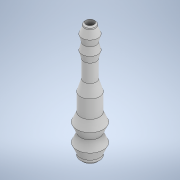
# Autodesk Inventor part: Barbed to Barbed 4mm ID to 2.4mm ID
Saved by Autodesk Inventor 2021 (Build 250183000, 183)
## iProperties
Created: 2020-12-17
Part Number: Barbed to Barbed 4mm ID to 2.4mm ID
Material: Generic
Document SubType Name: Modeling
Designer: natha
Density: 1 g/cm^3
Appearance: Default
Author: natha
Autodesk Inventor part; units mm, degrees
ref_plane "YZ Plane" through (0, 0, 0) normal (1, 0, 0) x (0, 1, 0)
ref_plane "XZ Plane" through (0, 0, 0) normal (0, 1, 0) x (-1, 0, 0)
ref_plane "XY Plane" through (0, 0, 0) normal (0, 0, 1) x (1, 0, 0)
sketch "Sketch1" plane through (0, 0, 0) normal (0, 0, 1) x (1, 0, 0)
  line L0 (-0.9, 16.5) -> (-0.9, -5.2047)
  line L1 (0, 21.8) -> (0, -15.3) construction
  line L2 (-0.9, 16.5) -> (-1.2, 16.2)
  line L3 (-1.2, 16.2) -> (-1.2, 15.9)
  line L4 (-1.2, 15.9) -> (-1.8, 14.3)
  line L5 (-1.8, 14.3) -> (-1.4, 12.7)
  line L6 (-1.4, 12.7) -> (-1.8, 11.1)
  line L7 (-1.8, 11.1) -> (-1.4, 9.5)
  line L8 (-1.4, 9.5) -> (-1.4, 5.5)
  line L9 (-1.4, 5.5) -> (-2.15, 3)
  line L10 (-2.15, 3) -> (-2.15, -1)
  line L11 (-2.15, -1) -> (-3, -3)
  line L12 (-3, -3) -> (-2.15, -5)
  line L13 (-2.15, -5) -> (-3, -7)
  line L14 (-3, -7) -> (-2.15, -9)
  line L15 (-2.15, -9) -> (-2.15, -9.5)
  line L16 (-2.15, -9.5) -> (-1.65, -10)
  line L17 (-1.65, -10) -> (-0.9, -10)
  line L18 (-0.9, -10) -> (-0.9, -5.2047)
  line L19 (-3.42, 0) -> (-0.48, 0) construction
  dimension "d5" = 0.9
  dimension "d6" = 1.8
  dimension "d15" = 1.2
  dimension "d16" = 1.8
  dimension "d18" = 45
  dimension "d19" = 0.3
  dimension "d20" = 1.4
  dimension "d21" = 1.4
  dimension "d22" = 1.6
  dimension "d23" = 1.6
  dimension "d24" = 1.6
  dimension "d27" = 4
  dimension "d29" = 2.5
  dimension "d30" = 2.15
  dimension "d31" = 4
  dimension "d32" = 1.6
  dimension "d33" = 2
  dimension "d34" = 2
  dimension "d35" = 2
  dimension "d36" = 2
  dimension "d37" = 3
  dimension "d38" = 2.15
  dimension "d39" = 3
  dimension "d41" = 45
  dimension "d42" = 0.5
  dimension "d43" = 0.5
  dimension "d44" = 10
  constraints: 36 end point, 4 vertical, 1 collinear, 1 parallel, 1 perpendicular
  measures "d5" distance between parallel lines of L1 L0
  measures "d6" distance from line of L1 L4.end
  measures "d15" distance between parallel lines of L1 L3
  measures "d16" distance from line of L1 L6.end
  measures "d18" angle of L1 L2
  measures "d19" distance of L2.end L3.end
  measures "d20" distance from line of L1 L5.end
  measures "d21" distance from line of L1 L7.end
  measures "d22" vertical distance of L4.end L3.end
  measures "d23" vertical distance of L7.end L6.end
  measures "d24" vertical distance of L6.end L5.end
  measures "d27" distance of L7.end L8.end
  measures "d29" vertical distance of L8.end L9.end
  measures "d30" distance from line of L1 L9.end
  measures "d31" distance of L9.end L10.end
  measures "d32" vertical distance of L5.end L4.end
  measures "d33" vertical distance of L10.end L11.end
  measures "d34" vertical distance of L11.end L12.end
  measures "d35" vertical distance of L12.end L13.end
  measures "d36" vertical distance of L13.end L14.end
  measures "d37" distance from line of L1 L11.end
  measures "d38" distance from line of L1 L12.end
  measures "d39" distance from line of L1 L13.end
  measures "d41" angle of L1 L16
  measures "d42" horizontal distance of L16.end L15.end
  measures "d43" distance of L14.end L15.end
  measures "d44" distance between parallel lines of L19 L17
revolve "Revolution1" add sketch "Sketch1" angle 360 about axis through (0, 0, 0) along (0, -1, 0)
equation "\"d23\" = d22"
equation "\"d24\" = d22"
equation "\"d32\" = d22"
equation "\"d34\" = d33"
equation "\"d35\" = d33"
equation "\"d36\" = d33"
equation "\"d38\" = d30"
equation "\"d39\" = d37"
body "Solid1"
